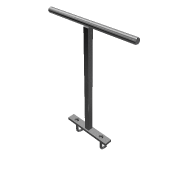
# Autodesk Inventor part: Schlüssel
Saved by Autodesk Inventor 2019 (Build 230136000, 136)
## iProperties
Created: 2016-08-28
Part Number: Schlüssel
Material: Stahl, galvanisiert
Document SubType Name: Modeling
Designer: Seelenernter
Density: 7.85 g/cm^3
Appearance: Stahl - galvanisiert
Author: Seelenernter
Autodesk Inventor part; units mm, degrees
ref_plane "XZ Plane" through (0, 0, 0) normal (0, 1, 0) x (-1, 0, 0)
sketch "Skizze1" plane through (0, 0, 0) normal (0, 0, 1) x (1, 0, 0)
  line L0 (10, -10) -> (-10, -10)
  line L1 (-10, -10) -> (-10, 10)
  line L2 (-10, 10) -> (10, 10)
  line L3 (10, 10) -> (10, -10)
  line L4 (10, -10) -> (-10, 10) construction
  line L5 (-10, -10) -> (10, 10) construction
  point P0 (0, 0)
  dimension "d0" = 20
  dimension "d1" = 20
  constraints: 12 end point, 2 midpoint, 2 parallel, 1 horizontal, 1 perpendicular
  measures "d0" distance of L1.end L2.end
  measures "d1" distance of L0.end L1.end
extrude "Extrusion1" add sketch "Skizze1" along normal blind 400
ref_plane "Arbeitsebene1" through (0, 0, 0) normal (1, 0, 0) x (0, 1, 0)
sketch "Skizze2" plane through (0, 0, 0) normal (1, 0, 0) x (0, 1, 0)
  line L0 (10, 0) -> (-10, 0) projected
  line L1 (10, 0) -> (10, 400) projected
  line L2 (-10, 400) -> (10, 400) projected
  line L3 (-10, 0) -> (-10, 400) projected
  circle A0 centre (0, 410) radius 10
  line L4 (-10, 400) -> (10, 400) projected
  point P0 (0, 0)
  point P1 (0, 400)
  dimension "d5" = 20
  constraints: 1 centre point, 1 midpoint, 1 tangent, 1 vertical alignment
  measures "d5" diameter of A0
extrude "Extrusion2" add sketch "Skizze2" along normal mid plane 350 contours A0
sketch "Skizze4" plane through (10, 10, 400) normal (1, 0, 0) x (0, 0, -1)
  circle A0 centre (-10, -10) radius 10 projected
  line L0 (400, 0) -> (400, -20) projected
  line L1 (400, 0) -> (0, 0) projected
  line L2 (0, -10) -> (0, 0) projected
  line L3 (0, -20) -> (0, -10) projected
  line L4 (400, -20) -> (0, -20) projected
  line L5 (0, -20) -> (0, -10) projected
  line L6 (0, -12.0268) -> (-0.2075, -12.0268)
  arc A1 (0, -20) -> (-3.0565, -17.1964) centre (-6.4849, -24.002) ccw
  circle A2 centre (-10, -10) radius 10 projected
  arc A3 (-3.0565, -17.1964) -> (-0.2075, -12.0268) centre (-10, -10) ccw
  line L7 (0, -20) -> (0, -12.0268)
  point P0 (400, -10)
  constraints: 4 end point, 4 point on circle, 2 centre point, 1 coincident, 1 collinear, 1 horizontal alignment, 1 perpendicular, 1 point on line, 2 other
extrude "Extrusion3" add sketch "Skizze4" against normal blind 20 contours A0 L6 L3 A1
mirror "Spiegeln1" about plane through (0, 0, 0) normal (0, 1, 0) of "Extrusion3"
fillet "Rundung1" radius 1 4 edges at (10, -10, 200) (-10, -10, 200) (-10, 10, 200) (10, 10, 200)
fillet "Rundung2" radius 3 2 edges at (175, -10, 410) (-175, -10, 410)
sketch "Skizze5" plane through (0, 0, 0) normal (0, 0, -1) x (-1, 0, 0)
  line L0 (-100, -15) -> (100, -15)
  line L1 (100, -15) -> (100, 15)
  line L2 (100, 15) -> (-100, 15)
  line L3 (-100, 15) -> (-100, -15)
  line L4 (-100, -15) -> (100, 15) construction
  line L5 (100, -15) -> (-100, 15) construction
  point P0 (0, 0)
  dimension "d12" = 30
  dimension "d13" = 200
  constraints: 12 end point, 2 midpoint, 2 parallel, 1 horizontal, 1 perpendicular
  measures "d12" distance of L2.end L0.start
  measures "d13" distance of L1.end L2.end
extrude "Extrusion4" add sketch "Skizze5" along normal blind 10
sketch "Skizze6" plane through (0, 0, 0) normal (0, 0, 1) x (1, 0, 0)
  line L0 (100, -15) -> (-100, -15) projected
  line L1 (100, 15) -> (100, -15) projected
  line L2 (-100, 15) -> (100, 15) projected
  line L3 (-100, -15) -> (-100, 15) projected
  arc A0 (-10, -9) -> (-9, -10) centre (-9, -9) ccw projected
  line L4 (-10, -9) -> (-10, 9) projected
  arc A1 (-9, 10) -> (-10, 9) centre (-9, 9) ccw projected
  line L5 (-9, 10) -> (9, 10) projected
  arc A2 (10, 9) -> (9, 10) centre (9, 9) ccw projected
  line L6 (10, 9) -> (10, -9) projected
  arc A3 (9, -10) -> (10, -9) centre (9, -9) ccw projected
  line L7 (9, -10) -> (-9, -10) projected
  circle A4 centre (65, 0) radius 5
  circle A5 centre (-65, 0) radius 5
  line L8 (10, 9) -> (10, -9) projected
  point P0 (0, 0)
  point P1 (10, 0)
  point P2 (-10, 0)
  dimension "d16" = 130
  dimension "d17" = 65
  dimension "d18" = 10
  dimension "d19" = 10
  constraints: 2 centre point, 2 horizontal alignment, 2 midpoint
  measures "d16" distance of A5.centre A4.centre
  measures "d17" distance of point (0, 0) A4.centre
  measures "d18" diameter of A4
  measures "d19" diameter of A5
extrude "Extrusion5" add sketch "Skizze6" along normal blind 10 contours A4 | A5
sketch "Skizze7" plane through (0, 0, -10) normal (0, 0, -1) x (-1, 0, 0)
  circle A0 centre (-65, 0) radius 5 projected
  circle A1 centre (65, 0) radius 5 projected
  point P0 (0, 0)
extrude "Extrusion6" add sketch "Skizze7" along normal blind 30
chamfer "Fase1" distance 4 angle 45 4 edges at (70, 0, -10) (60, 0, 0) (-70, 0, 0) (-60, 0, -10)
sketch "Skizze8" plane through (65, 0, -40) normal (0, 0, -1) x (-1, 0, 0)
  circle A0 centre (0, 0) radius 5 projected
  circle A1 centre (0, 0) radius 5 projected
  point P0 (65, 0)
ref_plane "Arbeitsebene2" through (65, 0, -40) normal (1, 0, 0) x (0, 0, -1)
sketch "Skizze9" plane through (65, 0, -40) normal (1, 0, 0) x (0, 0, -1)
  line L0 (-30, 15) -> (-30, -15) projected
  line L1 (0, -5) -> (0, 5) projected
  line L2 (0, 0) -> (10, 0)
  line L3 (30, 20) -> (30, 30)
  arc A0 (10, 0) -> (30, 20) centre (10, 20) ccw
  point P0 (-40, 0)
  point P1 (-30, 0)
  point P2 (30, 0)
  dimension "d29" = 30
  dimension "d30" = 30
  dimension "d31" = 20
  constraints: 4 end point, 2 midpoint, 2 point on circle, 2 point on line, 2 tangent, 1 centre point, 1 horizontal, 1 perpendicular
  measures "d29" distance of L2.start point (30, 0)
  measures "d30" distance of point (30, 0) L3.end
  measures "d31" radius of A0
sweep "Sweeping1" add profiles "Skizze8" path "Skizze9" path curves L2 A0 L3
mirror "Spiegeln2" about plane through (0, 0, 0) normal (1, 0, 0) of "Sweeping1"
